Autodesk Inventor part; units mm, degrees
(part 4 of 6)
  line L789 (-12.9119, -3.4916) -> (-26.3463, -3.4916)
  line L790 (-26.3463, -7.4916) -> (-12.9119, -7.4916)
  line L791 (-12.9119, -3.4916) -> (-26.3463, -3.4916)
  line L792 (-12.9119, -3.4916) -> (-26.3463, -3.4916)
  line L793 (-26.3463, -7.4916) -> (-12.9119, -7.4916)
  line L794 (-26.3463, -7.4916) -> (-12.9119, -7.4916)
  line L795 (-26.3463, -7.4916) -> (-12.9119, -7.4916)
  arc A894 (-12.9119, -7.4916) -> (-12.9119, -3.4916) centre (-12.9119, -5.4916) ccw
  arc A895 (-46.3463, -3.4916) -> (-46.3463, -7.4916) centre (-46.3463, -5.4916) ccw
  arc A896 (-52.9119, -7.4916) -> (-52.9119, -3.4916) centre (-52.9119, -5.4916) ccw
  arc A897 (-46.3463, -3.4916) -> (-46.3463, -7.4916) centre (-46.3463, -5.4916) ccw
  arc A898 (-46.3463, -3.4916) -> (-46.3463, -7.4916) centre (-46.3463, -5.4916) ccw
  arc A899 (-46.3463, -3.4916) -> (-46.3463, -7.4916) centre (-46.3463, -5.4916) ccw
  arc A900 (-46.3463, -3.4916) -> (-46.3463, -7.4916) centre (-46.3463, -5.4916) ccw
  arc A901 (-46.3463, -3.4916) -> (-46.3463, -7.4916) centre (-46.3463, -5.4916) ccw
  arc A902 (-52.9119, -7.4916) -> (-52.9119, -3.4916) centre (-52.9119, -5.4916) ccw
  arc A903 (-52.9119, -7.4916) -> (-52.9119, -3.4916) centre (-52.9119, -5.4916) ccw
  arc A904 (-52.9119, -7.4916) -> (-52.9119, -3.4916) centre (-52.9119, -5.4916) ccw
  arc A905 (-52.9119, -7.4916) -> (-52.9119, -3.4916) centre (-52.9119, -5.4916) ccw
  line L796 (-42.4124, 3.4654) -> (-55.8468, 3.4654)
  line L797 (-55.8468, -0.5346) -> (-42.4124, -0.5346)
  line L798 (-55.8468, -0.5346) -> (-42.4124, -0.5346)
  line L799 (-55.8468, -0.5346) -> (-42.4124, -0.5346)
  line L800 (-55.8468, -0.5346) -> (-42.4124, -0.5346)
  line L801 (-55.8468, -0.5346) -> (-42.4124, -0.5346)
  line L802 (-42.4124, 3.4654) -> (-55.8468, 3.4654)
  line L803 (-42.4124, 3.4654) -> (-55.8468, 3.4654)
  line L804 (-42.4124, 3.4654) -> (-55.8468, 3.4654)
  line L805 (-42.4124, 3.4654) -> (-55.8468, 3.4654)
  arc A906 (-86.3463, -3.4916) -> (-86.3463, -7.4916) centre (-86.3463, -5.4916) ccw
  arc A907 (-86.3463, -3.4916) -> (-86.3463, -7.4916) centre (-86.3463, -5.4916) ccw
  arc A908 (-86.3463, -3.4916) -> (-86.3463, -7.4916) centre (-86.3463, -5.4916) ccw
  arc A909 (-92.9119, -7.4916) -> (-92.9119, -3.4916) centre (-92.9119, -5.4916) ccw
  line L806 (-82.4124, 3.4654) -> (-95.8468, 3.4654)
  line L807 (-95.8468, -0.5346) -> (-82.4124, -0.5346)
  line L808 (-86.3463, -7.4916) -> (-72.9119, -7.4916)
  line L809 (-86.3463, -7.4916) -> (-72.9119, -7.4916)
  line L810 (-86.3463, -7.4916) -> (-72.9119, -7.4916)
  line L811 (-72.9119, -3.4916) -> (-86.3463, -3.4916)
  line L812 (-72.9119, -3.4916) -> (-86.3463, -3.4916)
  line L813 (-72.9119, -3.4916) -> (-86.3463, -3.4916)
  arc A910 (-75.8468, 3.4654) -> (-75.8468, -0.5346) centre (-75.8468, 1.4654) ccw
  arc A911 (-75.8468, 3.4654) -> (-75.8468, -0.5346) centre (-75.8468, 1.4654) ccw
  arc A912 (-75.8468, 3.4654) -> (-75.8468, -0.5346) centre (-75.8468, 1.4654) ccw
  arc A913 (-75.8468, 3.4654) -> (-75.8468, -0.5346) centre (-75.8468, 1.4654) ccw
  arc A914 (-82.4124, -0.5346) -> (-82.4124, 3.4654) centre (-82.4124, 1.4654) ccw
  line L814 (-66.3463, -7.4916) -> (-52.9119, -7.4916)
  line L815 (-52.9119, -3.4916) -> (-66.3463, -3.4916)
  line L816 (-52.9119, -3.4916) -> (-66.3463, -3.4916)
  line L817 (-66.3463, -7.4916) -> (-52.9119, -7.4916)
  line L818 (-52.9119, -3.4916) -> (-66.3463, -3.4916)
  line L819 (-52.9119, -3.4916) -> (-66.3463, -3.4916)
  line L820 (-52.9119, -3.4916) -> (-66.3463, -3.4916)
  line L821 (-66.3463, -7.4916) -> (-52.9119, -7.4916)
  line L822 (-66.3463, -7.4916) -> (-52.9119, -7.4916)
  line L823 (-66.3463, -7.4916) -> (-52.9119, -7.4916)
  line L824 (-46.3463, -7.4916) -> (-32.9119, -7.4916)
  line L825 (-32.9119, -3.4916) -> (-46.3463, -3.4916)
  line L826 (-32.9119, -3.4916) -> (-46.3463, -3.4916)
  line L827 (-46.3463, -7.4916) -> (-32.9119, -7.4916)
  line L828 (-32.9119, -3.4916) -> (-46.3463, -3.4916)
  line L829 (-32.9119, -3.4916) -> (-46.3463, -3.4916)
  line L830 (-32.9119, -3.4916) -> (-46.3463, -3.4916)
  line L831 (-46.3463, -7.4916) -> (-32.9119, -7.4916)
  line L832 (-46.3463, -7.4916) -> (-32.9119, -7.4916)
  line L833 (-46.3463, -7.4916) -> (-32.9119, -7.4916)
  line L834 (-46.3463, -7.4916) -> (-32.9119, -7.4916)
  line L835 (-32.9119, -3.4916) -> (-46.3463, -3.4916)
  arc A915 (-55.8468, 3.4654) -> (-55.8468, -0.5346) centre (-55.8468, 1.4654) ccw
  arc A916 (-55.8468, 3.4654) -> (-55.8468, -0.5346) centre (-55.8468, 1.4654) ccw
  arc A917 (-55.8468, 3.4654) -> (-55.8468, -0.5346) centre (-55.8468, 1.4654) ccw
  arc A918 (-62.4124, -0.5346) -> (-62.4124, 3.4654) centre (-62.4124, 1.4654) ccw
  arc A919 (-55.8468, 3.4654) -> (-55.8468, -0.5346) centre (-55.8468, 1.4654) ccw
  arc A920 (-55.8468, 3.4654) -> (-55.8468, -0.5346) centre (-55.8468, 1.4654) ccw
  arc A921 (-55.8468, 3.4654) -> (-55.8468, -0.5346) centre (-55.8468, 1.4654) ccw
  arc A922 (-55.8468, 3.4654) -> (-55.8468, -0.5346) centre (-55.8468, 1.4654) ccw
  arc A923 (-62.4124, -0.5346) -> (-62.4124, 3.4654) centre (-62.4124, 1.4654) ccw
  arc A924 (-62.4124, -0.5346) -> (-62.4124, 3.4654) centre (-62.4124, 1.4654) ccw
  arc A925 (-66.3463, -3.4916) -> (-66.3463, -7.4916) centre (-66.3463, -5.4916) ccw
  arc A926 (-72.9119, -7.4916) -> (-72.9119, -3.4916) centre (-72.9119, -5.4916) ccw
  arc A927 (-66.3463, -3.4916) -> (-66.3463, -7.4916) centre (-66.3463, -5.4916) ccw
  line L836 (-62.4124, 3.4654) -> (-75.8468, 3.4654)
  line L837 (-75.8468, -0.5346) -> (-62.4124, -0.5346)
  arc A928 (-72.9119, -7.4916) -> (-72.9119, -3.4916) centre (-72.9119, -5.4916) ccw
  line L838 (-62.4124, 3.4654) -> (-75.8468, 3.4654)
  line L839 (-75.8468, -0.5346) -> (-62.4124, -0.5346)
  arc A929 (-66.3463, -3.4916) -> (-66.3463, -7.4916) centre (-66.3463, -5.4916) ccw
  arc A930 (-66.3463, -3.4916) -> (-66.3463, -7.4916) centre (-66.3463, -5.4916) ccw
  arc A931 (-66.3463, -3.4916) -> (-66.3463, -7.4916) centre (-66.3463, -5.4916) ccw
  line L840 (-62.4124, 3.4654) -> (-75.8468, 3.4654)
  line L841 (-75.8468, -0.5346) -> (-62.4124, -0.5346)
  arc A932 (-72.9119, -7.4916) -> (-72.9119, -3.4916) centre (-72.9119, -5.4916) ccw
  arc A933 (-106.3463, -3.4916) -> (-106.3463, -7.4916) centre (-106.3463, -5.4916) ccw
  arc A934 (-95.8468, 3.4654) -> (-95.8468, -0.5346) centre (-95.8468, 1.4654) ccw
  line L842 (-92.9119, -3.4916) -> (-106.3463, -3.4916)
  line L843 (-106.3463, -7.4916) -> (-92.9119, -7.4916)
  arc A935 (-35.8468, 3.4654) -> (-35.8468, -0.5346) centre (-35.8468, 1.4654) ccw
  arc A936 (-35.8468, 3.4654) -> (-35.8468, -0.5346) centre (-35.8468, 1.4654) ccw
  arc A937 (-35.8468, 3.4654) -> (-35.8468, -0.5346) centre (-35.8468, 1.4654) ccw
  arc A938 (-42.4124, -0.5346) -> (-42.4124, 3.4654) centre (-42.4124, 1.4654) ccw
  arc A939 (-42.4124, -0.5346) -> (-42.4124, 3.4654) centre (-42.4124, 1.4654) ccw
  arc A940 (-35.8468, 3.4654) -> (-35.8468, -0.5346) centre (-35.8468, 1.4654) ccw
  arc A941 (-35.8468, 3.4654) -> (-35.8468, -0.5346) centre (-35.8468, 1.4654) ccw
  arc A942 (-35.8468, 3.4654) -> (-35.8468, -0.5346) centre (-35.8468, 1.4654) ccw
  arc A943 (-35.8468, 3.4654) -> (-35.8468, -0.5346) centre (-35.8468, 1.4654) ccw
  arc A944 (-35.8468, 3.4654) -> (-35.8468, -0.5346) centre (-35.8468, 1.4654) ccw
  arc A945 (-35.8468, 3.4654) -> (-35.8468, -0.5346) centre (-35.8468, 1.4654) ccw
  arc A946 (-42.4124, -0.5346) -> (-42.4124, 3.4654) centre (-42.4124, 1.4654) ccw
  arc A947 (-42.4124, -0.5346) -> (-42.4124, 3.4654) centre (-42.4124, 1.4654) ccw
  arc A948 (-42.4124, -0.5346) -> (-42.4124, 3.4654) centre (-42.4124, 1.4654) ccw
  arc A949 (44.1532, 17.4654) -> (44.1532, 13.4654) centre (44.1532, 15.4654) ccw
  arc A950 (44.1532, 17.4654) -> (44.1532, 13.4654) centre (44.1532, 15.4654) ccw
  arc A951 (44.1532, 17.4654) -> (44.1532, 13.4654) centre (44.1532, 15.4654) ccw
  arc A952 (44.1532, 17.4654) -> (44.1532, 13.4654) centre (44.1532, 15.4654) ccw
  arc A953 (44.1532, 17.4654) -> (44.1532, 13.4654) centre (44.1532, 15.4654) ccw
  arc A954 (44.1532, 17.4654) -> (44.1532, 13.4654) centre (44.1532, 15.4654) ccw
  arc A955 (44.1532, 17.4654) -> (44.1532, 13.4654) centre (44.1532, 15.4654) ccw
  arc A956 (33.6537, 10.5084) -> (33.6537, 6.5084) centre (33.6537, 8.5084) ccw
  arc A957 (27.0881, 6.5084) -> (27.0881, 10.5084) centre (27.0881, 8.5084) ccw
  arc A958 (27.0881, 6.5084) -> (27.0881, 10.5084) centre (27.0881, 8.5084) ccw
  arc A959 (33.6537, 10.5084) -> (33.6537, 6.5084) centre (33.6537, 8.5084) ccw
  arc A960 (27.0881, 6.5084) -> (27.0881, 10.5084) centre (27.0881, 8.5084) ccw
  arc A961 (27.0881, 6.5084) -> (27.0881, 10.5084) centre (27.0881, 8.5084) ccw
  arc A962 (27.0881, 6.5084) -> (27.0881, 10.5084) centre (27.0881, 8.5084) ccw
  arc A963 (27.0881, 6.5084) -> (27.0881, 10.5084) centre (27.0881, 8.5084) ccw
  arc A964 (33.6537, 10.5084) -> (33.6537, 6.5084) centre (33.6537, 8.5084) ccw
  arc A965 (33.6537, 10.5084) -> (33.6537, 6.5084) centre (33.6537, 8.5084) ccw
  arc A966 (33.6537, 10.5084) -> (33.6537, 6.5084) centre (33.6537, 8.5084) ccw
  line L844 (24.1532, 13.4654) -> (37.5876, 13.4654)
  line L845 (37.5876, 17.4654) -> (24.1532, 17.4654)
  line L846 (24.1532, 13.4654) -> (37.5876, 13.4654)
  line L847 (24.1532, 13.4654) -> (37.5876, 13.4654)
  line L848 (24.1532, 13.4654) -> (37.5876, 13.4654)
  line L849 (24.1532, 13.4654) -> (37.5876, 13.4654)
  line L850 (24.1532, 13.4654) -> (37.5876, 13.4654)
  line L851 (37.5876, 17.4654) -> (24.1532, 17.4654)
  line L852 (37.5876, 17.4654) -> (24.1532, 17.4654)
  line L853 (37.5876, 17.4654) -> (24.1532, 17.4654)
  line L854 (37.5876, 17.4654) -> (24.1532, 17.4654)
  line L855 (37.5876, 17.4654) -> (24.1532, 17.4654)
  arc A967 (37.5876, 13.4654) -> (37.5876, 17.4654) centre (37.5876, 15.4654) ccw
  arc A968 (37.5876, 13.4654) -> (37.5876, 17.4654) centre (37.5876, 15.4654) ccw
  arc A969 (37.5876, 13.4654) -> (37.5876, 17.4654) centre (37.5876, 15.4654) ccw
  arc A970 (37.5876, 13.4654) -> (37.5876, 17.4654) centre (37.5876, 15.4654) ccw
  arc A971 (37.5876, 13.4654) -> (37.5876, 17.4654) centre (37.5876, 15.4654) ccw
  arc A972 (37.5876, 13.4654) -> (37.5876, 17.4654) centre (37.5876, 15.4654) ccw
  arc A973 (44.1532, 17.4654) -> (44.1532, 13.4654) centre (44.1532, 15.4654) ccw
  arc A974 (47.0881, 6.5084) -> (47.0881, 10.5084) centre (47.0881, 8.5084) ccw
  arc A975 (47.0881, 6.5084) -> (47.0881, 10.5084) centre (47.0881, 8.5084) ccw
  arc A976 (53.6537, 10.5084) -> (53.6537, 6.5084) centre (53.6537, 8.5084) ccw
  arc A977 (47.0881, 6.5084) -> (47.0881, 10.5084) centre (47.0881, 8.5084) ccw
  arc A978 (47.0881, 6.5084) -> (47.0881, 10.5084) centre (47.0881, 8.5084) ccw
  arc A979 (47.0881, 6.5084) -> (47.0881, 10.5084) centre (47.0881, 8.5084) ccw
  arc A980 (53.6537, 10.5084) -> (53.6537, 6.5084) centre (53.6537, 8.5084) ccw
  arc A981 (53.6537, 10.5084) -> (53.6537, 6.5084) centre (53.6537, 8.5084) ccw
  line L856 (57.5876, 17.4654) -> (44.1532, 17.4654)
  line L857 (44.1532, 13.4654) -> (57.5876, 13.4654)
  line L858 (57.5876, 17.4654) -> (44.1532, 17.4654)
  line L859 (44.1532, 13.4654) -> (57.5876, 13.4654)
  line L860 (44.1532, 13.4654) -> (57.5876, 13.4654)
  line L861 (44.1532, 13.4654) -> (57.5876, 13.4654)
  line L862 (44.1532, 13.4654) -> (57.5876, 13.4654)
  line L863 (57.5876, 17.4654) -> (44.1532, 17.4654)
  line L864 (57.5876, 17.4654) -> (44.1532, 17.4654)
  line L865 (57.5876, 17.4654) -> (44.1532, 17.4654)
  arc A982 (57.5876, 13.4654) -> (57.5876, 17.4654) centre (57.5876, 15.4654) ccw
  arc A983 (64.1532, 17.4654) -> (64.1532, 13.4654) centre (64.1532, 15.4654) ccw
  line L866 (53.6537, 6.5084) -> (67.0881, 6.5084)
  line L867 (53.6537, 6.5084) -> (67.0881, 6.5084)
  line L868 (53.6537, 6.5084) -> (67.0881, 6.5084)
  line L869 (67.0881, 10.5084) -> (53.6537, 10.5084)
  line L870 (67.0881, 10.5084) -> (53.6537, 10.5084)
  line L871 (67.0881, 10.5084) -> (53.6537, 10.5084)
  arc A984 (64.1532, 17.4654) -> (64.1532, 13.4654) centre (64.1532, 15.4654) ccw
  arc A985 (64.1532, 17.4654) -> (64.1532, 13.4654) centre (64.1532, 15.4654) ccw
  arc A986 (64.1532, 17.4654) -> (64.1532, 13.4654) centre (64.1532, 15.4654) ccw
  arc A987 (64.1532, 17.4654) -> (64.1532, 13.4654) centre (64.1532, 15.4654) ccw
  arc A988 (57.5876, 13.4654) -> (57.5876, 17.4654) centre (57.5876, 15.4654) ccw
  arc A989 (57.5876, 13.4654) -> (57.5876, 17.4654) centre (57.5876, 15.4654) ccw
  arc A990 (57.5876, 13.4654) -> (57.5876, 17.4654) centre (57.5876, 15.4654) ccw
  arc A991 (57.5876, 13.4654) -> (57.5876, 17.4654) centre (57.5876, 15.4654) ccw
  arc A992 (67.0881, 6.5084) -> (67.0881, 10.5084) centre (67.0881, 8.5084) ccw
  arc A993 (67.0881, 6.5084) -> (67.0881, 10.5084) centre (67.0881, 8.5084) ccw
  arc A994 (67.0881, 6.5084) -> (67.0881, 10.5084) centre (67.0881, 8.5084) ccw
  line L872 (77.5876, 17.4654) -> (64.1532, 17.4654)
  line L873 (77.5876, 17.4654) -> (64.1532, 17.4654)
  line L874 (77.5876, 17.4654) -> (64.1532, 17.4654)
  line L875 (64.1532, 13.4654) -> (77.5876, 13.4654)
  line L876 (64.1532, 13.4654) -> (77.5876, 13.4654)
  line L877 (64.1532, 13.4654) -> (77.5876, 13.4654)
  arc A995 (73.6537, 10.5084) -> (73.6537, 6.5084) centre (73.6537, 8.5084) ccw
  arc A996 (77.5876, 13.4654) -> (77.5876, 17.4654) centre (77.5876, 15.4654) ccw
  arc A997 (77.5876, 13.4654) -> (77.5876, 17.4654) centre (77.5876, 15.4654) ccw
  arc A998 (77.5876, 13.4654) -> (77.5876, 17.4654) centre (77.5876, 15.4654) ccw
  arc A999 (84.1532, 17.4654) -> (84.1532, 13.4654) centre (84.1532, 15.4654) ccw
  arc A1000 (84.1532, 17.4654) -> (84.1532, 13.4654) centre (84.1532, 15.4654) ccw
  line L878 (87.0881, 10.5084) -> (73.6537, 10.5084)
  arc A1001 (87.0881, 6.5084) -> (87.0881, 10.5084) centre (87.0881, 8.5084) ccw
  line L879 (73.6537, 6.5084) -> (87.0881, 6.5084)
  line L880 (84.1532, 13.4654) -> (97.5876, 13.4654)
  line L881 (97.5876, 17.4654) -> (84.1532, 17.4654)
  arc A1002 (97.5876, 13.4654) -> (97.5876, 17.4654) centre (97.5876, 15.4654) ccw
  line L882 (33.6537, 6.5084) -> (47.0881, 6.5084)
  line L883 (47.0881, 10.5084) -> (33.6537, 10.5084)
  line L884 (33.6537, 6.5084) -> (47.0881, 6.5084)
  line L885 (47.0881, 10.5084) -> (33.6537, 10.5084)
  line L886 (47.0881, 10.5084) -> (33.6537, 10.5084)
  line L887 (47.0881, 10.5084) -> (33.6537, 10.5084)
  line L888 (47.0881, 10.5084) -> (33.6537, 10.5084)
  line L889 (33.6537, 6.5084) -> (47.0881, 6.5084)
  line L890 (33.6537, 6.5084) -> (47.0881, 6.5084)
  line L891 (33.6537, 6.5084) -> (47.0881, 6.5084)
  arc A1003 (13.6537, 10.5084) -> (13.6537, 6.5084) centre (13.6537, 8.5084) ccw
  arc A1004 (13.6537, 10.5084) -> (13.6537, 6.5084) centre (13.6537, 8.5084) ccw
  arc A1005 (13.6537, 10.5084) -> (13.6537, 6.5084) centre (13.6537, 8.5084) ccw
  arc A1006 (13.6537, 10.5084) -> (13.6537, 6.5084) centre (13.6537, 8.5084) ccw
  arc A1007 (13.6537, 10.5084) -> (13.6537, 6.5084) centre (13.6537, 8.5084) ccw
  arc A1008 (13.6537, 10.5084) -> (13.6537, 6.5084) centre (13.6537, 8.5084) ccw
  arc A1009 (7.0881, 6.5084) -> (7.0881, 10.5084) centre (7.0881, 8.5084) ccw
  arc A1010 (7.0881, 6.5084) -> (7.0881, 10.5084) centre (7.0881, 8.5084) ccw
  arc A1011 (7.0881, 6.5084) -> (7.0881, 10.5084) centre (7.0881, 8.5084) ccw
  arc A1012 (7.0881, 6.5084) -> (7.0881, 10.5084) centre (7.0881, 8.5084) ccw
  arc A1013 (17.5876, 13.4654) -> (17.5876, 17.4654) centre (17.5876, 15.4654) ccw
  arc A1014 (17.5876, 13.4654) -> (17.5876, 17.4654) centre (17.5876, 15.4654) ccw
  arc A1015 (17.5876, 13.4654) -> (17.5876, 17.4654) centre (17.5876, 15.4654) ccw
  arc A1016 (17.5876, 13.4654) -> (17.5876, 17.4654) centre (17.5876, 15.4654) ccw
  arc A1017 (17.5876, 13.4654) -> (17.5876, 17.4654) centre (17.5876, 15.4654) ccw
  arc A1018 (17.5876, 13.4654) -> (17.5876, 17.4654) centre (17.5876, 15.4654) ccw
  arc A1019 (24.1532, 17.4654) -> (24.1532, 13.4654) centre (24.1532, 15.4654) ccw
  arc A1020 (24.1532, 17.4654) -> (24.1532, 13.4654) centre (24.1532, 15.4654) ccw
  arc A1021 (24.1532, 17.4654) -> (24.1532, 13.4654) centre (24.1532, 15.4654) ccw
  arc A1022 (24.1532, 17.4654) -> (24.1532, 13.4654) centre (24.1532, 15.4654) ccw
  arc A1023 (24.1532, 17.4654) -> (24.1532, 13.4654) centre (24.1532, 15.4654) ccw
  arc A1024 (24.1532, 17.4654) -> (24.1532, 13.4654) centre (24.1532, 15.4654) ccw
  arc A1025 (24.1532, 17.4654) -> (24.1532, 13.4654) centre (24.1532, 15.4654) ccw
  arc A1026 (24.1532, 17.4654) -> (24.1532, 13.4654) centre (24.1532, 15.4654) ccw
  arc A1027 (24.1532, 17.4654) -> (24.1532, 13.4654) centre (24.1532, 15.4654) ccw
  arc A1028 (4.1532, 17.4654) -> (4.1532, 13.4654) centre (4.1532, 15.4654) ccw
  arc A1029 (4.1532, 17.4654) -> (4.1532, 13.4654) centre (4.1532, 15.4654) ccw
  arc A1030 (4.1532, 17.4654) -> (4.1532, 13.4654) centre (4.1532, 15.4654) ccw
  arc A1031 (4.1532, 17.4654) -> (4.1532, 13.4654) centre (4.1532, 15.4654) ccw
  arc A1032 (4.1532, 17.4654) -> (4.1532, 13.4654) centre (4.1532, 15.4654) ccw
  arc A1033 (4.1532, 17.4654) -> (4.1532, 13.4654) centre (4.1532, 15.4654) ccw
  arc A1034 (4.1532, 17.4654) -> (4.1532, 13.4654) centre (4.1532, 15.4654) ccw
  arc A1035 (4.1532, 17.4654) -> (4.1532, 13.4654) centre (4.1532, 15.4654) ccw
  arc A1036 (4.1532, 17.4654) -> (4.1532, 13.4654) centre (4.1532, 15.4654) ccw
  arc A1037 (-2.4124, 13.4654) -> (-2.4124, 17.4654) centre (-2.4124, 15.4654) ccw
  arc A1038 (-2.4124, 13.4654) -> (-2.4124, 17.4654) centre (-2.4124, 15.4654) ccw
  arc A1039 (-2.4124, 13.4654) -> (-2.4124, 17.4654) centre (-2.4124, 15.4654) ccw
  arc A1040 (-2.4124, 13.4654) -> (-2.4124, 17.4654) centre (-2.4124, 15.4654) ccw
  arc A1041 (-32.9119, 6.5084) -> (-32.9119, 10.5084) centre (-32.9119, 8.5084) ccw
  arc A1042 (-32.9119, 6.5084) -> (-32.9119, 10.5084) centre (-32.9119, 8.5084) ccw
  arc A1043 (-32.9119, 6.5084) -> (-32.9119, 10.5084) centre (-32.9119, 8.5084) ccw
  arc A1044 (-32.9119, 6.5084) -> (-32.9119, 10.5084) centre (-32.9119, 8.5084) ccw
  arc A1045 (-32.9119, 6.5084) -> (-32.9119, 10.5084) centre (-32.9119, 8.5084) ccw
  arc A1046 (-32.9119, 6.5084) -> (-32.9119, 10.5084) centre (-32.9119, 8.5084) ccw
  line L892 (27.0881, 10.5084) -> (13.6537, 10.5084)
  line L893 (13.6537, 6.5084) -> (27.0881, 6.5084)
  line L894 (27.0881, 10.5084) -> (13.6537, 10.5084)
  line L895 (13.6537, 6.5084) -> (27.0881, 6.5084)
  line L896 (13.6537, 6.5084) -> (27.0881, 6.5084)
  line L897 (27.0881, 10.5084) -> (13.6537, 10.5084)
  line L898 (27.0881, 10.5084) -> (13.6537, 10.5084)
  line L899 (27.0881, 10.5084) -> (13.6537, 10.5084)
  line L900 (13.6537, 6.5084) -> (27.0881, 6.5084)
  line L901 (13.6537, 6.5084) -> (27.0881, 6.5084)
  line L902 (13.6537, 6.5084) -> (27.0881, 6.5084)
  line L903 (27.0881, 10.5084) -> (13.6537, 10.5084)
  line L904 (4.1532, 13.4654) -> (17.5876, 13.4654)
  line L905 (4.1532, 13.4654) -> (17.5876, 13.4654)
  line L906 (4.1532, 13.4654) -> (17.5876, 13.4654)
  line L907 (4.1532, 13.4654) -> (17.5876, 13.4654)
  line L908 (4.1532, 13.4654) -> (17.5876, 13.4654)
  line L909 (4.1532, 13.4654) -> (17.5876, 13.4654)
  line L910 (17.5876, 17.4654) -> (4.1532, 17.4654)
  line L911 (17.5876, 17.4654) -> (4.1532, 17.4654)
  line L912 (17.5876, 17.4654) -> (4.1532, 17.4654)
  line L913 (17.5876, 17.4654) -> (4.1532, 17.4654)
  line L914 (17.5876, 17.4654) -> (4.1532, 17.4654)
  line L915 (17.5876, 17.4654) -> (4.1532, 17.4654)
  arc A1047 (7.0881, 6.5084) -> (7.0881, 10.5084) centre (7.0881, 8.5084) ccw
  arc A1048 (7.0881, 6.5084) -> (7.0881, 10.5084) centre (7.0881, 8.5084) ccw
  line L916 (-6.3463, 6.5084) -> (7.0881, 6.5084)
  line L917 (7.0881, 10.5084) -> (-6.3463, 10.5084)
  line L918 (7.0881, 10.5084) -> (-6.3463, 10.5084)
  line L919 (-6.3463, 6.5084) -> (7.0881, 6.5084)
  line L920 (-6.3463, 6.5084) -> (7.0881, 6.5084)
  line L921 (7.0881, 10.5084) -> (-6.3463, 10.5084)
  line L922 (7.0881, 10.5084) -> (-6.3463, 10.5084)
  line L923 (7.0881, 10.5084) -> (-6.3463, 10.5084)
  line L924 (-6.3463, 6.5084) -> (7.0881, 6.5084)
  line L925 (-6.3463, 6.5084) -> (7.0881, 6.5084)
  line L926 (-6.3463, 6.5084) -> (7.0881, 6.5084)
  line L927 (7.0881, 10.5084) -> (-6.3463, 10.5084)
  arc A1049 (-6.3463, 10.5084) -> (-6.3463, 6.5084) centre (-6.3463, 8.5084) ccw
  arc A1050 (-6.3463, 10.5084) -> (-6.3463, 6.5084) centre (-6.3463, 8.5084) ccw
  arc A1051 (-6.3463, 10.5084) -> (-6.3463, 6.5084) centre (-6.3463, 8.5084) ccw
  arc A1052 (-6.3463, 10.5084) -> (-6.3463, 6.5084) centre (-6.3463, 8.5084) ccw
  arc A1053 (-6.3463, 10.5084) -> (-6.3463, 6.5084) centre (-6.3463, 8.5084) ccw
  arc A1054 (-6.3463, 10.5084) -> (-6.3463, 6.5084) centre (-6.3463, 8.5084) ccw
  arc A1055 (-12.9119, 6.5084) -> (-12.9119, 10.5084) centre (-12.9119, 8.5084) ccw
  arc A1056 (-12.9119, 6.5084) -> (-12.9119, 10.5084) centre (-12.9119, 8.5084) ccw
  arc A1057 (-12.9119, 6.5084) -> (-12.9119, 10.5084) centre (-12.9119, 8.5084) ccw
  arc A1058 (-12.9119, 6.5084) -> (-12.9119, 10.5084) centre (-12.9119, 8.5084) ccw
  arc A1059 (-12.9119, 6.5084) -> (-12.9119, 10.5084) centre (-12.9119, 8.5084) ccw
  line L928 (-2.4124, 17.4654) -> (-15.8468, 17.4654)
  line L929 (-15.8468, 13.4654) -> (-2.4124, 13.4654)
  line L930 (-2.4124, 17.4654) -> (-15.8468, 17.4654)
  line L931 (-15.8468, 13.4654) -> (-2.4124, 13.4654)
  line L932 (-2.4124, 17.4654) -> (-15.8468, 17.4654)
  line L933 (-15.8468, 13.4654) -> (-2.4124, 13.4654)
  line L934 (-2.4124, 17.4654) -> (-15.8468, 17.4654)
  line L935 (-15.8468, 13.4654) -> (-2.4124, 13.4654)
  line L936 (-2.4124, 17.4654) -> (-15.8468, 17.4654)
  line L937 (-15.8468, 13.4654) -> (-2.4124, 13.4654)
  line L938 (-15.8468, 13.4654) -> (-2.4124, 13.4654)
  line L939 (-2.4124, 17.4654) -> (-15.8468, 17.4654)
  arc A1060 (-2.4124, 13.4654) -> (-2.4124, 17.4654) centre (-2.4124, 15.4654) ccw
  arc A1061 (-2.4124, 13.4654) -> (-2.4124, 17.4654) centre (-2.4124, 15.4654) ccw
  arc A1062 (-15.8468, 17.4654) -> (-15.8468, 13.4654) centre (-15.8468, 15.4654) ccw
  arc A1063 (-15.8468, 17.4654) -> (-15.8468, 13.4654) centre (-15.8468, 15.4654) ccw
  arc A1064 (-15.8468, 17.4654) -> (-15.8468, 13.4654) centre (-15.8468, 15.4654) ccw
  arc A1065 (-15.8468, 17.4654) -> (-15.8468, 13.4654) centre (-15.8468, 15.4654) ccw
  arc A1066 (-15.8468, 17.4654) -> (-15.8468, 13.4654) centre (-15.8468, 15.4654) ccw
  arc A1067 (-22.4124, 13.4654) -> (-22.4124, 17.4654) centre (-22.4124, 15.4654) ccw
  arc A1068 (-22.4124, 13.4654) -> (-22.4124, 17.4654) centre (-22.4124, 15.4654) ccw
  arc A1069 (-15.8468, 17.4654) -> (-15.8468, 13.4654) centre (-15.8468, 15.4654) ccw
  arc A1070 (-15.8468, 17.4654) -> (-15.8468, 13.4654) centre (-15.8468, 15.4654) ccw
  arc A1071 (-22.4124, 13.4654) -> (-22.4124, 17.4654) centre (-22.4124, 15.4654) ccw
  arc A1072 (-15.8468, 17.4654) -> (-15.8468, 13.4654) centre (-15.8468, 15.4654) ccw
  arc A1073 (-15.8468, 17.4654) -> (-15.8468, 13.4654) centre (-15.8468, 15.4654) ccw
  arc A1074 (-22.4124, 13.4654) -> (-22.4124, 17.4654) centre (-22.4124, 15.4654) ccw
  arc A1075 (-22.4124, 13.4654) -> (-22.4124, 17.4654) centre (-22.4124, 15.4654) ccw
  arc A1076 (-22.4124, 13.4654) -> (-22.4124, 17.4654) centre (-22.4124, 15.4654) ccw
  arc A1077 (-26.3463, 10.5084) -> (-26.3463, 6.5084) centre (-26.3463, 8.5084) ccw
  arc A1078 (-26.3463, 10.5084) -> (-26.3463, 6.5084) centre (-26.3463, 8.5084) ccw
  arc A1079 (-26.3463, 10.5084) -> (-26.3463, 6.5084) centre (-26.3463, 8.5084) ccw
  arc A1080 (-26.3463, 10.5084) -> (-26.3463, 6.5084) centre (-26.3463, 8.5084) ccw
  arc A1081 (-26.3463, 10.5084) -> (-26.3463, 6.5084) centre (-26.3463, 8.5084) ccw
  arc A1082 (-26.3463, 10.5084) -> (-26.3463, 6.5084) centre (-26.3463, 8.5084) ccw
  line L940 (-35.8468, 13.4654) -> (-22.4124, 13.4654)
  line L941 (-35.8468, 13.4654) -> (-22.4124, 13.4654)
  line L942 (-35.8468, 13.4654) -> (-22.4124, 13.4654)
  line L943 (-35.8468, 13.4654) -> (-22.4124, 13.4654)
  line L944 (-35.8468, 13.4654) -> (-22.4124, 13.4654)
  line L945 (-35.8468, 13.4654) -> (-22.4124, 13.4654)
  line L946 (-22.4124, 17.4654) -> (-35.8468, 17.4654)
  line L947 (-22.4124, 17.4654) -> (-35.8468, 17.4654)
  line L948 (-22.4124, 17.4654) -> (-35.8468, 17.4654)
  line L949 (-22.4124, 17.4654) -> (-35.8468, 17.4654)
  line L950 (-22.4124, 17.4654) -> (-35.8468, 17.4654)
  line L951 (-22.4124, 17.4654) -> (-35.8468, 17.4654)
  line L952 (-26.3463, 6.5084) -> (-12.9119, 6.5084)
  line L953 (-12.9119, 10.5084) -> (-26.3463, 10.5084)
  line L954 (-12.9119, 10.5084) -> (-26.3463, 10.5084)
  line L955 (-26.3463, 6.5084) -> (-12.9119, 6.5084)
  line L956 (-12.9119, 10.5084) -> (-26.3463, 10.5084)
  line L957 (-12.9119, 10.5084) -> (-26.3463, 10.5084)
  line L958 (-26.3463, 6.5084) -> (-12.9119, 6.5084)
  line L959 (-12.9119, 10.5084) -> (-26.3463, 10.5084)
  line L960 (-12.9119, 10.5084) -> (-26.3463, 10.5084)
  line L961 (-26.3463, 6.5084) -> (-12.9119, 6.5084)
  line L962 (-26.3463, 6.5084) -> (-12.9119, 6.5084)
  line L963 (-26.3463, 6.5084) -> (-12.9119, 6.5084)
  arc A1083 (-12.9119, 6.5084) -> (-12.9119, 10.5084) centre (-12.9119, 8.5084) ccw
  arc A1084 (-46.3463, 10.5084) -> (-46.3463, 6.5084) centre (-46.3463, 8.5084) ccw
  arc A1085 (-52.9119, 6.5084) -> (-52.9119, 10.5084) centre (-52.9119, 8.5084) ccw
  arc A1086 (-46.3463, 10.5084) -> (-46.3463, 6.5084) centre (-46.3463, 8.5084) ccw
  arc A1087 (-46.3463, 10.5084) -> (-46.3463, 6.5084) centre (-46.3463, 8.5084) ccw
  arc A1088 (-46.3463, 10.5084) -> (-46.3463, 6.5084) centre (-46.3463, 8.5084) ccw
  arc A1089 (-46.3463, 10.5084) -> (-46.3463, 6.5084) centre (-46.3463, 8.5084) ccw
  arc A1090 (-46.3463, 10.5084) -> (-46.3463, 6.5084) centre (-46.3463, 8.5084) ccw
  arc A1091 (-52.9119, 6.5084) -> (-52.9119, 10.5084) centre (-52.9119, 8.5084) ccw
  arc A1092 (-52.9119, 6.5084) -> (-52.9119, 10.5084) centre (-52.9119, 8.5084) ccw
  arc A1093 (-52.9119, 6.5084) -> (-52.9119, 10.5084) centre (-52.9119, 8.5084) ccw
  arc A1094 (-52.9119, 6.5084) -> (-52.9119, 10.5084) centre (-52.9119, 8.5084) ccw
  line L964 (-42.4124, 17.4654) -> (-55.8468, 17.4654)
  line L965 (-55.8468, 13.4654) -> (-42.4124, 13.4654)
  line L966 (-55.8468, 13.4654) -> (-42.4124, 13.4654)
  line L967 (-55.8468, 13.4654) -> (-42.4124, 13.4654)
  line L968 (-55.8468, 13.4654) -> (-42.4124, 13.4654)
  line L969 (-55.8468, 13.4654) -> (-42.4124, 13.4654)
  line L970 (-42.4124, 17.4654) -> (-55.8468, 17.4654)
  line L971 (-42.4124, 17.4654) -> (-55.8468, 17.4654)
  line L972 (-42.4124, 17.4654) -> (-55.8468, 17.4654)
  line L973 (-42.4124, 17.4654) -> (-55.8468, 17.4654)
  arc A1095 (-86.3463, 10.5084) -> (-86.3463, 6.5084) centre (-86.3463, 8.5084) ccw
  arc A1096 (-86.3463, 10.5084) -> (-86.3463, 6.5084) centre (-86.3463, 8.5084) ccw
  arc A1097 (-86.3463, 10.5084) -> (-86.3463, 6.5084) centre (-86.3463, 8.5084) ccw
  arc A1098 (-92.9119, 6.5084) -> (-92.9119, 10.5084) centre (-92.9119, 8.5084) ccw
  line L974 (-82.4124, 17.4654) -> (-95.8468, 17.4654)
  line L975 (-95.8468, 13.4654) -> (-82.4124, 13.4654)
  line L976 (-86.3463, 6.5084) -> (-72.9119, 6.5084)
  line L977 (-86.3463, 6.5084) -> (-72.9119, 6.5084)
  line L978 (-86.3463, 6.5084) -> (-72.9119, 6.5084)
  line L979 (-72.9119, 10.5084) -> (-86.3463, 10.5084)
  line L980 (-72.9119, 10.5084) -> (-86.3463, 10.5084)
  line L981 (-72.9119, 10.5084) -> (-86.3463, 10.5084)
  arc A1099 (-75.8468, 17.4654) -> (-75.8468, 13.4654) centre (-75.8468, 15.4654) ccw
  arc A1100 (-75.8468, 17.4654) -> (-75.8468, 13.4654) centre (-75.8468, 15.4654) ccw
  arc A1101 (-75.8468, 17.4654) -> (-75.8468, 13.4654) centre (-75.8468, 15.4654) ccw
  arc A1102 (-75.8468, 17.4654) -> (-75.8468, 13.4654) centre (-75.8468, 15.4654) ccw
  arc A1103 (-82.4124, 13.4654) -> (-82.4124, 17.4654) centre (-82.4124, 15.4654) ccw
  line L982 (-66.3463, 6.5084) -> (-52.9119, 6.5084)
  line L983 (-52.9119, 10.5084) -> (-66.3463, 10.5084)
  line L984 (-52.9119, 10.5084) -> (-66.3463, 10.5084)
  line L985 (-66.3463, 6.5084) -> (-52.9119, 6.5084)
  line L986 (-52.9119, 10.5084) -> (-66.3463, 10.5084)
  line L987 (-52.9119, 10.5084) -> (-66.3463, 10.5084)
  line L988 (-52.9119, 10.5084) -> (-66.3463, 10.5084)
  line L989 (-66.3463, 6.5084) -> (-52.9119, 6.5084)
  line L990 (-66.3463, 6.5084) -> (-52.9119, 6.5084)
  line L991 (-66.3463, 6.5084) -> (-52.9119, 6.5084)
  line L992 (-46.3463, 6.5084) -> (-32.9119, 6.5084)
  line L993 (-32.9119, 10.5084) -> (-46.3463, 10.5084)
  line L994 (-32.9119, 10.5084) -> (-46.3463, 10.5084)
  line L995 (-46.3463, 6.5084) -> (-32.9119, 6.5084)
  line L996 (-32.9119, 10.5084) -> (-46.3463, 10.5084)
  line L997 (-32.9119, 10.5084) -> (-46.3463, 10.5084)
  line L998 (-32.9119, 10.5084) -> (-46.3463, 10.5084)
  line L999 (-46.3463, 6.5084) -> (-32.9119, 6.5084)
  line L1000 (-46.3463, 6.5084) -> (-32.9119, 6.5084)
  line L1001 (-46.3463, 6.5084) -> (-32.9119, 6.5084)
  line L1002 (-46.3463, 6.5084) -> (-32.9119, 6.5084)
  line L1003 (-32.9119, 10.5084) -> (-46.3463, 10.5084)
  arc A1104 (-55.8468, 17.4654) -> (-55.8468, 13.4654) centre (-55.8468, 15.4654) ccw
  arc A1105 (-55.8468, 17.4654) -> (-55.8468, 13.4654) centre (-55.8468, 15.4654) ccw
  arc A1106 (-55.8468, 17.4654) -> (-55.8468, 13.4654) centre (-55.8468, 15.4654) ccw
  arc A1107 (-62.4124, 13.4654) -> (-62.4124, 17.4654) centre (-62.4124, 15.4654) ccw
  arc A1108 (-55.8468, 17.4654) -> (-55.8468, 13.4654) centre (-55.8468, 15.4654) ccw
  arc A1109 (-55.8468, 17.4654) -> (-55.8468, 13.4654) centre (-55.8468, 15.4654) ccw
  arc A1110 (-55.8468, 17.4654) -> (-55.8468, 13.4654) centre (-55.8468, 15.4654) ccw
  arc A1111 (-55.8468, 17.4654) -> (-55.8468, 13.4654) centre (-55.8468, 15.4654) ccw
  arc A1112 (-62.4124, 13.4654) -> (-62.4124, 17.4654) centre (-62.4124, 15.4654) ccw
  arc A1113 (-62.4124, 13.4654) -> (-62.4124, 17.4654) centre (-62.4124, 15.4654) ccw
  arc A1114 (-66.3463, 10.5084) -> (-66.3463, 6.5084) centre (-66.3463, 8.5084) ccw
  arc A1115 (-72.9119, 6.5084) -> (-72.9119, 10.5084) centre (-72.9119, 8.5084) ccw
  arc A1116 (-66.3463, 10.5084) -> (-66.3463, 6.5084) centre (-66.3463, 8.5084) ccw
  line L1004 (-62.4124, 17.4654) -> (-75.8468, 17.4654)
  line L1005 (-75.8468, 13.4654) -> (-62.4124, 13.4654)
  arc A1117 (-72.9119, 6.5084) -> (-72.9119, 10.5084) centre (-72.9119, 8.5084) ccw
  line L1006 (-62.4124, 17.4654) -> (-75.8468, 17.4654)
  line L1007 (-75.8468, 13.4654) -> (-62.4124, 13.4654)
  arc A1118 (-66.3463, 10.5084) -> (-66.3463, 6.5084) centre (-66.3463, 8.5084) ccw
  arc A1119 (-66.3463, 10.5084) -> (-66.3463, 6.5084) centre (-66.3463, 8.5084) ccw
  arc A1120 (-66.3463, 10.5084) -> (-66.3463, 6.5084) centre (-66.3463, 8.5084) ccw
  line L1008 (-62.4124, 17.4654) -> (-75.8468, 17.4654)
  line L1009 (-75.8468, 13.4654) -> (-62.4124, 13.4654)
  arc A1121 (-72.9119, 6.5084) -> (-72.9119, 10.5084) centre (-72.9119, 8.5084) ccw
  arc A1122 (-106.3463, 10.5084) -> (-106.3463, 6.5084) centre (-106.3463, 8.5084) ccw
  arc A1123 (-95.8468, 17.4654) -> (-95.8468, 13.4654) centre (-95.8468, 15.4654) ccw
  line L1010 (-92.9119, 10.5084) -> (-106.3463, 10.5084)
  line L1011 (-106.3463, 6.5084) -> (-92.9119, 6.5084)
  arc A1124 (-35.8468, 17.4654) -> (-35.8468, 13.4654) centre (-35.8468, 15.4654) ccw
  arc A1125 (-35.8468, 17.4654) -> (-35.8468, 13.4654) centre (-35.8468, 15.4654) ccw
  arc A1126 (-35.8468, 17.4654) -> (-35.8468, 13.4654) centre (-35.8468, 15.4654) ccw
  arc A1127 (-42.4124, 13.4654) -> (-42.4124, 17.4654) centre (-42.4124, 15.4654) ccw
  arc A1128 (-42.4124, 13.4654) -> (-42.4124, 17.4654) centre (-42.4124, 15.4654) ccw
  arc A1129 (-35.8468, 17.4654) -> (-35.8468, 13.4654) centre (-35.8468, 15.4654) ccw
  arc A1130 (-35.8468, 17.4654) -> (-35.8468, 13.4654) centre (-35.8468, 15.4654) ccw
  arc A1131 (-35.8468, 17.4654) -> (-35.8468, 13.4654) centre (-35.8468, 15.4654) ccw
  arc A1132 (-35.8468, 17.4654) -> (-35.8468, 13.4654) centre (-35.8468, 15.4654) ccw
  arc A1133 (-35.8468, 17.4654) -> (-35.8468, 13.4654) centre (-35.8468, 15.4654) ccw
  arc A1134 (-35.8468, 17.4654) -> (-35.8468, 13.4654) centre (-35.8468, 15.4654) ccw
  arc A1135 (-42.4124, 13.4654) -> (-42.4124, 17.4654) centre (-42.4124, 15.4654) ccw
  arc A1136 (-42.4124, 13.4654) -> (-42.4124, 17.4654) centre (-42.4124, 15.4654) ccw
  arc A1137 (-42.4124, 13.4654) -> (-42.4124, 17.4654) centre (-42.4124, 15.4654) ccw
  arc A1138 (44.1532, 31.4654) -> (44.1532, 27.4654) centre (44.1532, 29.4654) ccw
  arc A1139 (44.1532, 31.4654) -> (44.1532, 27.4654) centre (44.1532, 29.4654) ccw
  arc A1140 (44.1532, 31.4654) -> (44.1532, 27.4654) centre (44.1532, 29.4654) ccw
  arc A1141 (44.1532, 31.4654) -> (44.1532, 27.4654) centre (44.1532, 29.4654) ccw
  arc A1142 (44.1532, 31.4654) -> (44.1532, 27.4654) centre (44.1532, 29.4654) ccw
  arc A1143 (44.1532, 31.4654) -> (44.1532, 27.4654) centre (44.1532, 29.4654) ccw
  arc A1144 (44.1532, 31.4654) -> (44.1532, 27.4654) centre (44.1532, 29.4654) ccw
  arc A1145 (33.6537, 24.5084) -> (33.6537, 20.5084) centre (33.6537, 22.5084) ccw
  arc A1146 (27.0881, 20.5084) -> (27.0881, 24.5084) centre (27.0881, 22.5084) ccw
  arc A1147 (27.0881, 20.5084) -> (27.0881, 24.5084) centre (27.0881, 22.5084) ccw
  arc A1148 (33.6537, 24.5084) -> (33.6537, 20.5084) centre (33.6537, 22.5084) ccw
  arc A1149 (27.0881, 20.5084) -> (27.0881, 24.5084) centre (27.0881, 22.5084) ccw
  arc A1150 (27.0881, 20.5084) -> (27.0881, 24.5084) centre (27.0881, 22.5084) ccw
  arc A1151 (27.0881, 20.5084) -> (27.0881, 24.5084) centre (27.0881, 22.5084) ccw
  arc A1152 (27.0881, 20.5084) -> (27.0881, 24.5084) centre (27.0881, 22.5084) ccw
  arc A1153 (33.6537, 24.5084) -> (33.6537, 20.5084) centre (33.6537, 22.5084) ccw
  arc A1154 (33.6537, 24.5084) -> (33.6537, 20.5084) centre (33.6537, 22.5084) ccw
  arc A1155 (33.6537, 24.5084) -> (33.6537, 20.5084) centre (33.6537, 22.5084) ccw
  line L1012 (24.1532, 27.4654) -> (37.5876, 27.4654)
  line L1013 (37.5876, 31.4654) -> (24.1532, 31.4654)
  line L1014 (24.1532, 27.4654) -> (37.5876, 27.4654)
  line L1015 (24.1532, 27.4654) -> (37.5876, 27.4654)
  line L1016 (24.1532, 27.4654) -> (37.5876, 27.4654)
  line L1017 (24.1532, 27.4654) -> (37.5876, 27.4654)
  line L1018 (24.1532, 27.4654) -> (37.5876, 27.4654)
  line L1019 (37.5876, 31.4654) -> (24.1532, 31.4654)
  line L1020 (37.5876, 31.4654) -> (24.1532, 31.4654)
  line L1021 (37.5876, 31.4654) -> (24.1532, 31.4654)
  line L1022 (37.5876, 31.4654) -> (24.1532, 31.4654)
  line L1023 (37.5876, 31.4654) -> (24.1532, 31.4654)
  arc A1156 (37.5876, 27.4654) -> (37.5876, 31.4654) centre (37.5876, 29.4654) ccw
  arc A1157 (37.5876, 27.4654) -> (37.5876, 31.4654) centre (37.5876, 29.4654) ccw
  arc A1158 (37.5876, 27.4654) -> (37.5876, 31.4654) centre (37.5876, 29.4654) ccw
  arc A1159 (37.5876, 27.4654) -> (37.5876, 31.4654) centre (37.5876, 29.4654) ccw
  arc A1160 (37.5876, 27.4654) -> (37.5876, 31.4654) centre (37.5876, 29.4654) ccw
  arc A1161 (37.5876, 27.4654) -> (37.5876, 31.4654) centre (37.5876, 29.4654) ccw
  arc A1162 (44.1532, 31.4654) -> (44.1532, 27.4654) centre (44.1532, 29.4654) ccw
  arc A1163 (47.0881, 20.5084) -> (47.0881, 24.5084) centre (47.0881, 22.5084) ccw
  arc A1164 (47.0881, 20.5084) -> (47.0881, 24.5084) centre (47.0881, 22.5084) ccw
  arc A1165 (53.6537, 24.5084) -> (53.6537, 20.5084) centre (53.6537, 22.5084) ccw
  arc A1166 (47.0881, 20.5084) -> (47.0881, 24.5084) centre (47.0881, 22.5084) ccw
  arc A1167 (47.0881, 20.5084) -> (47.0881, 24.5084) centre (47.0881, 22.5084) ccw
  arc A1168 (47.0881, 20.5084) -> (47.0881, 24.5084) centre (47.0881, 22.5084) ccw
  arc A1169 (53.6537, 24.5084) -> (53.6537, 20.5084) centre (53.6537, 22.5084) ccw
  arc A1170 (53.6537, 24.5084) -> (53.6537, 20.5084) centre (53.6537, 22.5084) ccw
  line L1024 (57.5876, 31.4654) -> (44.1532, 31.4654)
  line L1025 (44.1532, 27.4654) -> (57.5876, 27.4654)
  line L1026 (57.5876, 31.4654) -> (44.1532, 31.4654)
  line L1027 (44.1532, 27.4654) -> (57.5876, 27.4654)
  line L1028 (44.1532, 27.4654) -> (57.5876, 27.4654)
  line L1029 (44.1532, 27.4654) -> (57.5876, 27.4654)
  line L1030 (44.1532, 27.4654) -> (57.5876, 27.4654)
  line L1031 (57.5876, 31.4654) -> (44.1532, 31.4654)
  line L1032 (57.5876, 31.4654) -> (44.1532, 31.4654)
  line L1033 (57.5876, 31.4654) -> (44.1532, 31.4654)
  arc A1171 (57.5876, 27.4654) -> (57.5876, 31.4654) centre (57.5876, 29.4654) ccw
  arc A1172 (64.1532, 31.4654) -> (64.1532, 27.4654) centre (64.1532, 29.4654) ccw
  line L1034 (53.6537, 20.5084) -> (67.0881, 20.5084)
  line L1035 (53.6537, 20.5084) -> (67.0881, 20.5084)
  line L1036 (53.6537, 20.5084) -> (67.0881, 20.5084)
  line L1037 (67.0881, 24.5084) -> (53.6537, 24.5084)
  line L1038 (67.0881, 24.5084) -> (53.6537, 24.5084)
  line L1039 (67.0881, 24.5084) -> (53.6537, 24.5084)
  arc A1173 (64.1532, 31.4654) -> (64.1532, 27.4654) centre (64.1532, 29.4654) ccw
  arc A1174 (64.1532, 31.4654) -> (64.1532, 27.4654) centre (64.1532, 29.4654) ccw
  arc A1175 (64.1532, 31.4654) -> (64.1532, 27.4654) centre (64.1532, 29.4654) ccw
  arc A1176 (64.1532, 31.4654) -> (64.1532, 27.4654) centre (64.1532, 29.4654) ccw
  arc A1177 (57.5876, 27.4654) -> (57.5876, 31.4654) centre (57.5876, 29.4654) ccw
  arc A1178 (57.5876, 27.4654) -> (57.5876, 31.4654) centre (57.5876, 29.4654) ccw
  arc A1179 (57.5876, 27.4654) -> (57.5876, 31.4654) centre (57.5876, 29.4654) ccw
  arc A1180 (57.5876, 27.4654) -> (57.5876, 31.4654) centre (57.5876, 29.4654) ccw
  arc A1181 (67.0881, 20.5084) -> (67.0881, 24.5084) centre (67.0881, 22.5084) ccw
  arc A1182 (67.0881, 20.5084) -> (67.0881, 24.5084) centre (67.0881, 22.5084) ccw
  arc A1183 (67.0881, 20.5084) -> (67.0881, 24.5084) centre (67.0881, 22.5084) ccw
  line L1040 (77.5876, 31.4654) -> (64.1532, 31.4654)
  line L1041 (77.5876, 31.4654) -> (64.1532, 31.4654)
  line L1042 (77.5876, 31.4654) -> (64.1532, 31.4654)
  line L1043 (64.1532, 27.4654) -> (77.5876, 27.4654)
  line L1044 (64.1532, 27.4654) -> (77.5876, 27.4654)
  line L1045 (64.1532, 27.4654) -> (77.5876, 27.4654)
  arc A1184 (73.6537, 24.5084) -> (73.6537, 20.5084) centre (73.6537, 22.5084) ccw
  arc A1185 (77.5876, 27.4654) -> (77.5876, 31.4654) centre (77.5876, 29.4654) ccw
  arc A1186 (77.5876, 27.4654) -> (77.5876, 31.4654) centre (77.5876, 29.4654) ccw
  arc A1187 (77.5876, 27.4654) -> (77.5876, 31.4654) centre (77.5876, 29.4654) ccw
  arc A1188 (84.1532, 31.4654) -> (84.1532, 27.4654) centre (84.1532, 29.4654) ccw
  arc A1189 (84.1532, 31.4654) -> (84.1532, 27.4654) centre (84.1532, 29.4654) ccw
  line L1046 (87.0881, 24.5084) -> (73.6537, 24.5084)
  arc A1190 (87.0881, 20.5084) -> (87.0881, 24.5084) centre (87.0881, 22.5084) ccw
  line L1047 (73.6537, 20.5084) -> (87.0881, 20.5084)
  line L1048 (84.1532, 27.4654) -> (97.5876, 27.4654)
  line L1049 (97.5876, 31.4654) -> (84.1532, 31.4654)
  arc A1191 (97.5876, 27.4654) -> (97.5876, 31.4654) centre (97.5876, 29.4654) ccw
  line L1050 (33.6537, 20.5084) -> (47.0881, 20.5084)
  line L1051 (47.0881, 24.5084) -> (33.6537, 24.5084)
  line L1052 (33.6537, 20.5084) -> (47.0881, 20.5084)
  line L1053 (47.0881, 24.5084) -> (33.6537, 24.5084)
  line L1054 (47.0881, 24.5084) -> (33.6537, 24.5084)
  line L1055 (47.0881, 24.5084) -> (33.6537, 24.5084)
  line L1056 (47.0881, 24.5084) -> (33.6537, 24.5084)
  line L1057 (33.6537, 20.5084) -> (47.0881, 20.5084)
  line L1058 (33.6537, 20.5084) -> (47.0881, 20.5084)
  line L1059 (33.6537, 20.5084) -> (47.0881, 20.5084)
  arc A1192 (13.6537, 24.5084) -> (13.6537, 20.5084) centre (13.6537, 22.5084) ccw
  arc A1193 (13.6537, 24.5084) -> (13.6537, 20.5084) centre (13.6537, 22.5084) ccw
  arc A1194 (13.6537, 24.5084) -> (13.6537, 20.5084) centre (13.6537, 22.5084) ccw
  arc A1195 (13.6537, 24.5084) -> (13.6537, 20.5084) centre (13.6537, 22.5084) ccw
  arc A1196 (13.6537, 24.5084) -> (13.6537, 20.5084) centre (13.6537, 22.5084) ccw
  arc A1197 (13.6537, 24.5084) -> (13.6537, 20.5084) centre (13.6537, 22.5084) ccw
  arc A1198 (7.0881, 20.5084) -> (7.0881, 24.5084) centre (7.0881, 22.5084) ccw
  arc A1199 (7.0881, 20.5084) -> (7.0881, 24.5084) centre (7.0881, 22.5084) ccw
  arc A1200 (7.0881, 20.5084) -> (7.0881, 24.5084) centre (7.0881, 22.5084) ccw
  arc A1201 (7.0881, 20.5084) -> (7.0881, 24.5084) centre (7.0881, 22.5084) ccw
  arc A1202 (17.5876, 27.4654) -> (17.5876, 31.4654) centre (17.5876, 29.4654) ccw
  arc A1203 (17.5876, 27.4654) -> (17.5876, 31.4654) centre (17.5876, 29.4654) ccw
  arc A1204 (17.5876, 27.4654) -> (17.5876, 31.4654) centre (17.5876, 29.4654) ccw
  arc A1205 (17.5876, 27.4654) -> (17.5876, 31.4654) centre (17.5876, 29.4654) ccw
  arc A1206 (17.5876, 27.4654) -> (17.5876, 31.4654) centre (17.5876, 29.4654) ccw
  arc A1207 (17.5876, 27.4654) -> (17.5876, 31.4654) centre (17.5876, 29.4654) ccw
  arc A1208 (24.1532, 31.4654) -> (24.1532, 27.4654) centre (24.1532, 29.4654) ccw
  arc A1209 (24.1532, 31.4654) -> (24.1532, 27.4654) centre (24.1532, 29.4654) ccw
  arc A1210 (24.1532, 31.4654) -> (24.1532, 27.4654) centre (24.1532, 29.4654) ccw
  arc A1211 (24.1532, 31.4654) -> (24.1532, 27.4654) centre (24.1532, 29.4654) ccw
  arc A1212 (24.1532, 31.4654) -> (24.1532, 27.4654) centre (24.1532, 29.4654) ccw
  arc A1213 (24.1532, 31.4654) -> (24.1532, 27.4654) centre (24.1532, 29.4654) ccw
  arc A1214 (24.1532, 31.4654) -> (24.1532, 27.4654) centre (24.1532, 29.4654) ccw
  arc A1215 (24.1532, 31.4654) -> (24.1532, 27.4654) centre (24.1532, 29.4654) ccw
  arc A1216 (24.1532, 31.4654) -> (24.1532, 27.4654) centre (24.1532, 29.4654) ccw
  arc A1217 (4.1532, 31.4654) -> (4.1532, 27.4654) centre (4.1532, 29.4654) ccw
  arc A1218 (4.1532, 31.4654) -> (4.1532, 27.4654) centre (4.1532, 29.4654) ccw
  arc A1219 (4.1532, 31.4654) -> (4.1532, 27.4654) centre (4.1532, 29.4654) ccw
  arc A1220 (4.1532, 31.4654) -> (4.1532, 27.4654) centre (4.1532, 29.4654) ccw
  arc A1221 (4.1532, 31.4654) -> (4.1532, 27.4654) centre (4.1532, 29.4654) ccw
  arc A1222 (4.1532, 31.4654) -> (4.1532, 27.4654) centre (4.1532, 29.4654) ccw
  arc A1223 (4.1532, 31.4654) -> (4.1532, 27.4654) centre (4.1532, 29.4654) ccw
  arc A1224 (4.1532, 31.4654) -> (4.1532, 27.4654) centre (4.1532, 29.4654) ccw
  arc A1225 (4.1532, 31.4654) -> (4.1532, 27.4654) centre (4.1532, 29.4654) ccw
  arc A1226 (-2.4124, 27.4654) -> (-2.4124, 31.4654) centre (-2.4124, 29.4654) ccw
  arc A1227 (-2.4124, 27.4654) -> (-2.4124, 31.4654) centre (-2.4124, 29.4654) ccw
  arc A1228 (-2.4124, 27.4654) -> (-2.4124, 31.4654) centre (-2.4124, 29.4654) ccw
  arc A1229 (-2.4124, 27.4654) -> (-2.4124, 31.4654) centre (-2.4124, 29.4654) ccw
  arc A1230 (-32.9119, 20.5084) -> (-32.9119, 24.5084) centre (-32.9119, 22.5084) ccw
  arc A1231 (-32.9119, 20.5084) -> (-32.9119, 24.5084) centre (-32.9119, 22.5084) ccw
  arc A1232 (-32.9119, 20.5084) -> (-32.9119, 24.5084) centre (-32.9119, 22.5084) ccw
  arc A1233 (-32.9119, 20.5084) -> (-32.9119, 24.5084) centre (-32.9119, 22.5084) ccw
  arc A1234 (-32.9119, 20.5084) -> (-32.9119, 24.5084) centre (-32.9119, 22.5084) ccw
  arc A1235 (-32.9119, 20.5084) -> (-32.9119, 24.5084) centre (-32.9119, 22.5084) ccw
  line L1060 (27.0881, 24.5084) -> (13.6537, 24.5084)
  line L1061 (13.6537, 20.5084) -> (27.0881, 20.5084)
  line L1062 (27.0881, 24.5084) -> (13.6537, 24.5084)
  line L1063 (13.6537, 20.5084) -> (27.0881, 20.5084)
  line L1064 (13.6537, 20.5084) -> (27.0881, 20.5084)
  line L1065 (27.0881, 24.5084) -> (13.6537, 24.5084)
  line L1066 (27.0881, 24.5084) -> (13.6537, 24.5084)
  line L1067 (27.0881, 24.5084) -> (13.6537, 24.5084)
  line L1068 (13.6537, 20.5084) -> (27.0881, 20.5084)
  line L1069 (13.6537, 20.5084) -> (27.0881, 20.5084)
  line L1070 (13.6537, 20.5084) -> (27.0881, 20.5084)
  line L1071 (27.0881, 24.5084) -> (13.6537, 24.5084)
  line L1072 (4.1532, 27.4654) -> (17.5876, 27.4654)
  line L1073 (4.1532, 27.4654) -> (17.5876, 27.4654)
  line L1074 (4.1532, 27.4654) -> (17.5876, 27.4654)
  line L1075 (4.1532, 27.4654) -> (17.5876, 27.4654)
  line L1076 (4.1532, 27.4654) -> (17.5876, 27.4654)
  line L1077 (4.1532, 27.4654) -> (17.5876, 27.4654)
  line L1078 (17.5876, 31.4654) -> (4.1532, 31.4654)
  line L1079 (17.5876, 31.4654) -> (4.1532, 31.4654)
  line L1080 (17.5876, 31.4654) -> (4.1532, 31.4654)
  line L1081 (17.5876, 31.4654) -> (4.1532, 31.4654)
  line L1082 (17.5876, 31.4654) -> (4.1532, 31.4654)
  line L1083 (17.5876, 31.4654) -> (4.1532, 31.4654)
  arc A1236 (7.0881, 20.5084) -> (7.0881, 24.5084) centre (7.0881, 22.5084) ccw
  arc A1237 (7.0881, 20.5084) -> (7.0881, 24.5084) centre (7.0881, 22.5084) ccw
  line L1084 (-6.3463, 20.5084) -> (7.0881, 20.5084)
  line L1085 (7.0881, 24.5084) -> (-6.3463, 24.5084)
  line L1086 (7.0881, 24.5084) -> (-6.3463, 24.5084)
  line L1087 (-6.3463, 20.5084) -> (7.0881, 20.5084)
  line L1088 (-6.3463, 20.5084) -> (7.0881, 20.5084)
  line L1089 (7.0881, 24.5084) -> (-6.3463, 24.5084)
  line L1090 (7.0881, 24.5084) -> (-6.3463, 24.5084)
  line L1091 (7.0881, 24.5084) -> (-6.3463, 24.5084)
  line L1092 (-6.3463, 20.5084) -> (7.0881, 20.5084)
  line L1093 (-6.3463, 20.5084) -> (7.0881, 20.5084)
  line L1094 (-6.3463, 20.5084) -> (7.0881, 20.5084)
  line L1095 (7.0881, 24.5084) -> (-6.3463, 24.5084)
  arc A1238 (-6.3463, 24.5084) -> (-6.3463, 20.5084) centre (-6.3463, 22.5084) ccw
  arc A1239 (-6.3463, 24.5084) -> (-6.3463, 20.5084) centre (-6.3463, 22.5084) ccw
  arc A1240 (-6.3463, 24.5084) -> (-6.3463, 20.5084) centre (-6.3463, 22.5084) ccw
  arc A1241 (-6.3463, 24.5084) -> (-6.3463, 20.5084) centre (-6.3463, 22.5084) ccw
  arc A1242 (-6.3463, 24.5084) -> (-6.3463, 20.5084) centre (-6.3463, 22.5084) ccw
  arc A1243 (-6.3463, 24.5084) -> (-6.3463, 20.5084) centre (-6.3463, 22.5084) ccw
  arc A1244 (-12.9119, 20.5084) -> (-12.9119, 24.5084) centre (-12.9119, 22.5084) ccw
  arc A1245 (-12.9119, 20.5084) -> (-12.9119, 24.5084) centre (-12.9119, 22.5084) ccw
  arc A1246 (-12.9119, 20.5084) -> (-12.9119, 24.5084) centre (-12.9119, 22.5084) ccw
  arc A1247 (-12.9119, 20.5084) -> (-12.9119, 24.5084) centre (-12.9119, 22.5084) ccw
  arc A1248 (-12.9119, 20.5084) -> (-12.9119, 24.5084) centre (-12.9119, 22.5084) ccw
  line L1096 (-2.4124, 31.4654) -> (-15.8468, 31.4654)
  line L1097 (-15.8468, 27.4654) -> (-2.4124, 27.4654)
  line L1098 (-2.4124, 31.4654) -> (-15.8468, 31.4654)
  line L1099 (-15.8468, 27.4654) -> (-2.4124, 27.4654)
  line L1100 (-2.4124, 31.4654) -> (-15.8468, 31.4654)
  line L1101 (-15.8468, 27.4654) -> (-2.4124, 27.4654)
  line L1102 (-2.4124, 31.4654) -> (-15.8468, 31.4654)
  line L1103 (-15.8468, 27.4654) -> (-2.4124, 27.4654)
  line L1104 (-2.4124, 31.4654) -> (-15.8468, 31.4654)
  line L1105 (-15.8468, 27.4654) -> (-2.4124, 27.4654)
  line L1106 (-15.8468, 27.4654) -> (-2.4124, 27.4654)
  line L1107 (-2.4124, 31.4654) -> (-15.8468, 31.4654)
  arc A1249 (-2.4124, 27.4654) -> (-2.4124, 31.4654) centre (-2.4124, 29.4654) ccw
  arc A1250 (-2.4124, 27.4654) -> (-2.4124, 31.4654) centre (-2.4124, 29.4654) ccw
  arc A1251 (-15.8468, 31.4654) -> (-15.8468, 27.4654) centre (-15.8468, 29.4654) ccw
  arc A1252 (-15.8468, 31.4654) -> (-15.8468, 27.4654) centre (-15.8468, 29.4654) ccw
  arc A1253 (-15.8468, 31.4654) -> (-15.8468, 27.4654) centre (-15.8468, 29.4654) ccw
  arc A1254 (-15.8468, 31.4654) -> (-15.8468, 27.4654) centre (-15.8468, 29.4654) ccw
  arc A1255 (-15.8468, 31.4654) -> (-15.8468, 27.4654) centre (-15.8468, 29.4654) ccw
  arc A1256 (-22.4124, 27.4654) -> (-22.4124, 31.4654) centre (-22.4124, 29.4654) ccw
  arc A1257 (-22.4124, 27.4654) -> (-22.4124, 31.4654) centre (-22.4124, 29.4654) ccw
  arc A1258 (-15.8468, 31.4654) -> (-15.8468, 27.4654) centre (-15.8468, 29.4654) ccw
  arc A1259 (-15.8468, 31.4654) -> (-15.8468, 27.4654) centre (-15.8468, 29.4654) ccw
  arc A1260 (-22.4124, 27.4654) -> (-22.4124, 31.4654) centre (-22.4124, 29.4654) ccw
  arc A1261 (-15.8468, 31.4654) -> (-15.8468, 27.4654) centre (-15.8468, 29.4654) ccw
  arc A1262 (-15.8468, 31.4654) -> (-15.8468, 27.4654) centre (-15.8468, 29.4654) ccw
  arc A1263 (-22.4124, 27.4654) -> (-22.4124, 31.4654) centre (-22.4124, 29.4654) ccw
  arc A1264 (-22.4124, 27.4654) -> (-22.4124, 31.4654) centre (-22.4124, 29.4654) ccw
  arc A1265 (-22.4124, 27.4654) -> (-22.4124, 31.4654) centre (-22.4124, 29.4654) ccw
  arc A1266 (-26.3463, 24.5084) -> (-26.3463, 20.5084) centre (-26.3463, 22.5084) ccw
  arc A1267 (-26.3463, 24.5084) -> (-26.3463, 20.5084) centre (-26.3463, 22.5084) ccw
  arc A1268 (-26.3463, 24.5084) -> (-26.3463, 20.5084) centre (-26.3463, 22.5084) ccw
  arc A1269 (-26.3463, 24.5084) -> (-26.3463, 20.5084) centre (-26.3463, 22.5084) ccw
  arc A1270 (-26.3463, 24.5084) -> (-26.3463, 20.5084) centre (-26.3463, 22.5084) ccw
  arc A1271 (-26.3463, 24.5084) -> (-26.3463, 20.5084) centre (-26.3463, 22.5084) ccw
  line L1108 (-35.8468, 27.4654) -> (-22.4124, 27.4654)
  line L1109 (-35.8468, 27.4654) -> (-22.4124, 27.4654)
  line L1110 (-35.8468, 27.4654) -> (-22.4124, 27.4654)
  line L1111 (-35.8468, 27.4654) -> (-22.4124, 27.4654)
  line L1112 (-35.8468, 27.4654) -> (-22.4124, 27.4654)
  line L1113 (-35.8468, 27.4654) -> (-22.4124, 27.4654)
  line L1114 (-22.4124, 31.4654) -> (-35.8468, 31.4654)
  line L1115 (-22.4124, 31.4654) -> (-35.8468, 31.4654)
  line L1116 (-22.4124, 31.4654) -> (-35.8468, 31.4654)
  line L1117 (-22.4124, 31.4654) -> (-35.8468, 31.4654)
  line L1118 (-22.4124, 31.4654) -> (-35.8468, 31.4654)
  line L1119 (-22.4124, 31.4654) -> (-35.8468, 31.4654)
  line L1120 (-26.3463, 20.5084) -> (-12.9119, 20.5084)
  line L1121 (-12.9119, 24.5084) -> (-26.3463, 24.5084)
  line L1122 (-12.9119, 24.5084) -> (-26.3463, 24.5084)
  line L1123 (-26.3463, 20.5084) -> (-12.9119, 20.5084)
  line L1124 (-12.9119, 24.5084) -> (-26.3463, 24.5084)
  line L1125 (-12.9119, 24.5084) -> (-26.3463, 24.5084)
  line L1126 (-26.3463, 20.5084) -> (-12.9119, 20.5084)
  line L1127 (-12.9119, 24.5084) -> (-26.3463, 24.5084)
  line L1128 (-12.9119, 24.5084) -> (-26.3463, 24.5084)
  line L1129 (-26.3463, 20.5084) -> (-12.9119, 20.5084)
  line L1130 (-26.3463, 20.5084) -> (-12.9119, 20.5084)